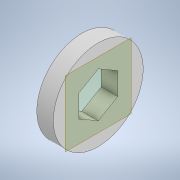
# Autodesk Inventor part: wheel_gearing_mount_extension
Saved by Autodesk Inventor 2021 (Build 250183000, 183)
## iProperties
Created: 2021-01-28
Part Number: wheel_gearing_mount_extension
Material: Generic
Document SubType Name: Modeling
Designer: Mateusz
Density: 1 g/cm^3
Appearance: Default
Author: Mateusz
Autodesk Inventor part; units mm, degrees
ref_plane "YZ Plane" through (0, 0, 0) normal (1, 0, 0) x (0, 1, 0)
ref_plane "XZ Plane" through (0, 0, 0) normal (0, 1, 0) x (-1, 0, 0)
ref_plane "XY Plane" through (0, 0, 0) normal (0, 0, 1) x (1, 0, 0)
ref_plane "Work Plane1" through (0, 0, 0) normal (-1, 0, 0) x (0, 0, 1)
sketch "Sketch1" plane through (0, 0, 0) normal (-1, 0, 0) x (0, 0, 1)
  circle A0 centre (0, 0) radius 15 projected
  line L0 (-6.4952, 3.75) -> (-6.4952, -3.75) projected
  line L1 (0, 7.5) -> (-6.4952, 3.75) projected
  line L2 (6.4952, 3.75) -> (0, 7.5) projected
  line L3 (6.4952, -3.75) -> (6.4952, 3.75) projected
  line L4 (0, -7.5) -> (6.4952, -3.75) projected
  line L5 (-6.4952, -3.75) -> (0, -7.5) projected
extrude "Extrusion1" add sketch "Sketch1" along normal blind 5.5
body "Solid2"
